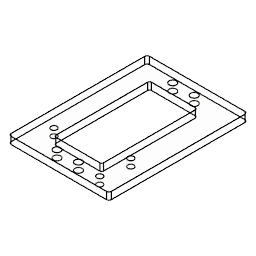
ServoPlate_v4 (Autodesk Fusion 360 design; units mm, degrees)
Autodesk Fusion 360 part; units mm, degrees
sketch "Sketch1" plane through (0, 0, 0) normal (0, 0, 1) x (1, 0, 0)
  line L0 (-10, 20) -> (10, 20)
  circle A0 centre (-4.5, 24.24) radius 1.5
  line L1 (0, 24.24) -> (0, 20) construction
  circle A1 centre (4.5, 24.24) radius 1.5
  line L2 (4.5, 24.24) -> (-4.5, 24.24) construction
  line L3 (0, 0) -> (10.6295, 0) construction
  line L4 (0, 0) -> (0, 5.1011) construction
  line L5 (10, -20) -> (-10, -20)
  line L6 (10, 20) -> (10, -20)
  line L7 (-10, -20) -> (10, 20) construction
  line L8 (22, -29) -> (22, 29)
  line L9 (-10, -20) -> (-10, 20)
  line L10 (10, -20) -> (-10, 20) construction
  line L11 (-20, -29) -> (-20, 29)
  line L12 (22, 29) -> (-20, 29)
  line L13 (22, -29) -> (-20, -29)
  circle A2 centre (-4.5, -24.24) radius 1.5
  circle A3 centre (4.5, -24.24) radius 1.5
  circle A4 centre (-13, -17) radius 1.25
  circle A5 centre (-13, -17) radius 2.5 construction
  line L14 (-10, -20) -> (-13, -20) construction
  line L15 (-13, -20) -> (-13, -17) construction
  line L16 (-10.5, -17) -> (-10, -17) construction
  line L17 (-15.5, -17) -> (-20, -17) construction
  line L18 (-10.5, -17) -> (-13, -17) construction
  circle A6 centre (14.1, -24.9) radius 1.25
  line L19 (14.1, -24.9) -> (14.1, -11.9) construction
  circle A7 centre (14.1, -11.9) radius 1.25
  circle A8 centre (14.1, -11.9) radius 4.1 construction
  circle A9 centre (14.1, -24.9) radius 4.1 construction
  dimension "d3" = 20
  dimension "d4" = 40
  dimension "d6" = 9
  dimension "d8" = 4.24
  dimension "d9" = 3
  dimension "d10" = 3
  dimension "d18" = 9
  dimension "d19" = 10
  dimension "d20" = 12
  dimension "d21" = 2.5
  dimension "d22" = 5
  dimension "d23" = 3
  dimension "d26" = 3
  dimension "d29" = 0.5
  dimension "d31" = 4.5
  dimension "d32" = 2.5
  dimension "d33" = 2.5
  dimension "d34" = 13
  dimension "d35" = 8.2
  dimension "d36" = 8.2
  constraint coincident L3.start L4.start
  constraint horizontal L5
  constraint perpendicular L5 L9
  constraint parallel L0 L5
  constraint parallel L6 L9
  constraint coincident L3.start L10
  constraint coincident L3.start L7
  constraint coincident L4.start L3
  constraint midpoint L1.start L2
  constraint coincident L1.end L0
  constraint perpendicular L0 L1
  constraint midpoint L1.end L0
  constraint perpendicular L1 L2
  constraint vertical L4
  constraint vertical L8
  constraint vertical L11
  constraint perpendicular L11 L12
  constraint coincident A0.centre L2.end
  constraint coincident A1.centre L2.start
  constraint symmetric L11.end L3 L11.start
  constraint symmetric L8.end L3 L8.start
  constraint symmetric A0 L3 A2
  constraint symmetric A1 L3 A3
  constraint perpendicular L9 L14
  constraint coincident A4.centre A5.centre
  constraint perpendicular L14 L15
  constraint coincident A5 L16.start
  constraint coincident L9 L16.end
  constraint perpendicular L9 L16
  constraint coincident A5 L17.start
  constraint horizontal L17
  constraint collinear L16 L17
  constraint horizontal L18
  constraint coincident L11 L17.end
  constraint coincident A6.centre L19.start
  constraint vertical L19
  constraint coincident L19.end A7.centre
  constraint concentric A7 A8
  constraint concentric A6 A9
  constraint tangent L6 A8
  constraint tangent L13 A9
  measures "d3" distance of L0.start L0.end
  measures "d4" distance of L0.start L5.end
  measures "d6" distance of A0.centre A1.centre
  measures "d8" distance of L1.end L1.start
  measures "d9" diameter of A1
  measures "d10" diameter of A0
  measures "d18" distance of L0 L12
  measures "d19" distance of L9 L11
  measures "d20" distance of L6 L8
  measures "d21" diameter of A4
  measures "d22" diameter of A5
  measures "d23" distance of L5.end L14.end
  measures "d26" distance of L14.end A4.centre
  measures "d29" distance of L16.start L16.end
  measures "d31" distance of L17.start L17.end
  measures "d32" diameter of A6
  measures "d33" diameter of A7
  measures "d34" distance of A6.centre L19.end
  measures "d35" diameter of A8
  measures "d36" diameter of A9
extrude "Extrude1" add sketch "Sketch1" along normal blind 3
fillet "Fillet1" radius 0.75 4 edges at (-10, -20, 1.5) (10, -20, 1.5) (10, 20, 1.5) (-10, 20, 1.5)
fillet "Fillet2" radius 1 4 edges at (-20, -29, 1.5) (22, -29, 1.5) (-20, 29, 1.5) (22, 29, 1.5)
sketch "Laser" plane through (0, 0, 3) normal (0, 0, 1) x (-1, 0, 0)
  arc A0 (-22, -28) -> (-21, -29) centre (-21, -28) ccw
  line L0 (-21, -29) -> (19, -29)
  arc A1 (19, -29) -> (20, -28) centre (19, -28) ccw
  line L1 (20, -28) -> (20, 28)
  arc A2 (20, 28) -> (19, 29) centre (19, 28) ccw
  line L2 (19, 29) -> (-21, 29)
  arc A3 (-21, 29) -> (-22, 28) centre (-21, 28) ccw
  line L3 (-22, 28) -> (-22, -28)
  circle A4 centre (-14.1, 11.9) radius 1.25
  circle A5 centre (4.5, -24.24) radius 1.5
  circle A6 centre (4.5, 24.24) radius 1.5
  circle A7 centre (13, 17) radius 1.25
  circle A8 centre (-4.5, 24.24) radius 1.5
  circle A9 centre (-14.1, 24.9) radius 1.25
  line L4 (-9.25, 20) -> (9.25, 20)
  arc A10 (10, 19.25) -> (9.25, 20) centre (9.25, 19.25) ccw
  line L5 (10, 19.25) -> (10, -19.25)
  arc A11 (9.25, -20) -> (10, -19.25) centre (9.25, -19.25) ccw
  line L6 (9.25, -20) -> (-9.25, -20)
  arc A12 (-10, -19.25) -> (-9.25, -20) centre (-9.25, -19.25) ccw
  line L7 (-10, -19.25) -> (-10, 19.25)
  arc A13 (-9.25, 20) -> (-10, 19.25) centre (-9.25, 19.25) ccw
  circle A14 centre (-4.5, -24.24) radius 1.5
  line L8 (-14.1, 11.9) -> (-14.1, 24.9) construction
  line L9 (-16, 22) -> (-12.2, 22)
  line L10 (-12.2, 22) -> (-12.2, 14.8)
  line L11 (-12.2, 14.8) -> (-16, 14.8)
  line L12 (-16, 14.8) -> (-16, 22)
  line L13 (-16, 22) -> (-12.2, 14.8) construction
  line L14 (-12.2, 22) -> (-16, 14.8) construction
  point P0 (-14.1, 18.4)
  constraint coincident A4.centre L8.start
  constraint coincident A9.centre L8.end
  constraint horizontal L9
  constraint perpendicular L9 L10
  constraint parallel L9 L11
  constraint parallel L10 L12
  constraint coincident L13 P0
  constraint coincident L14 P0
  constraint midpoint L8 P0
equation "d20 = 8 mm + 4 mm"
